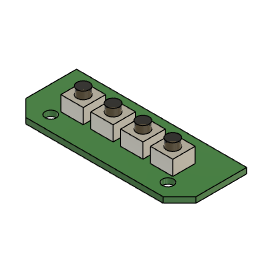
Tamabunni v1 (Autodesk Fusion 360 archive; units mm, degrees)
design "button_pad"
Autodesk Fusion 360 part; units mm, degrees
sketch "Sketch1" plane through (0, 0, 0) normal (0, 0, 1) x (1, 0, 0)
  line L0 (-22.8, 10) -> (22.8, 10)
  line L1 (22.8, 10) -> (22.8, -10)
  line L2 (22.8, -10) -> (-22.8, -10)
  line L3 (-22.8, -10) -> (-22.8, 10)
  line L4 (-22.8, 10) -> (22.8, -10) construction
  line L5 (-15, 4) -> (-9, 4)
  line L6 (-9, 4) -> (-9, -2)
  line L7 (-9, -2) -> (-15, -2)
  line L8 (-15, -2) -> (-15, 4)
  line L9 (0, 10) -> (0, -10) construction
  line L10 (-1, -2) -> (-7, -2)
  line L11 (-7, -2) -> (-7, 4)
  line L12 (-7, 4) -> (-1, 4)
  line L13 (-1, 4) -> (-1, -2)
  line L14 (7, 4) -> (1, 4)
  line L15 (1, 4) -> (1, -2)
  line L16 (1, -2) -> (7, -2)
  line L17 (7, -2) -> (7, 4)
  line L18 (15, 4) -> (9, 4)
  line L19 (9, 4) -> (9, -2)
  line L20 (15, -2) -> (15, 4)
  line L21 (9, -2) -> (15, -2)
  circle A0 centre (-15.7, -4) radius 1.5
  circle A1 centre (15.7, -4) radius 1.5
  line L22 (-15.7, -4) -> (15.7, -4) construction
  dimension "d1" = 45.6
  dimension "d2" = 20
  dimension "d3" = 6
  dimension "d4" = 6
  dimension "d5" = 2
  dimension "d6" = 1
  dimension "d7" = 6
  dimension "d33" = 7.1
  dimension "d34" = 3
  dimension "d37" = 3
  dimension "d38" = 6
  dimension "d59" = 7.1
  constraint horizontal L0
  constraint vertical L1
  constraint horizontal L2
  constraint vertical L3
  constraint midpoint origin L4
  constraint horizontal L5
  constraint vertical L6
  constraint horizontal L7
  constraint vertical L8
  constraint equal L5 L6
  constraint midpoint L0 L9.start
  constraint midpoint L2 L9.end
  constraint horizontal L12
  constraint vertical L13
  constraint horizontal L10
  constraint vertical L11
  constraint equal L12 L13
  constraint collinear L5 L12
  constraint symmetric L5.start L9 L18.start
  constraint symmetric L5.end L9 L18.end
  constraint symmetric L6.end L9 L19.end
  constraint symmetric L7.end L9 L20.start
  constraint symmetric L9 L10.start L15.end
  constraint symmetric L9 L11.end L14.start
  constraint symmetric L9 L10.end L16.end
  constraint symmetric L9 L12.end L14.end
  constraint coincident A0.centre L22.start
  constraint coincident A1.centre L22.end
  constraint horizontal L22
  measures "d1" distance of L0.start L0.end
  measures "d2" distance of L0.start L2.end
  measures "d3" distance of L5.end L6.end
  measures "d4" distance of L10.start L12.end
  measures "d5" distance of L6 L11
  measures "d6" distance of L9 L13
  measures "d7" distance of L0 L12
  measures "d33" distance of L1 A1.centre
  measures "d34" diameter of A1
  measures "d37" diameter of A0
  measures "d38" distance of L2 A1.centre
  measures "d59" distance of L3 A0.centre
extrude "Extrude7" add sketch "Sketch1" against normal blind 1.5 contours L0 L1 L2 L3 | L5 L6 L7 L8 | L10 L11 L12 L13 | L14 L15 L16 L17 | L18 L19 L20 L21
extrude "Extrude8" add sketch "Sketch1" along normal blind 4 contours L5 L6 L7 L8 | L10 L11 L12 L13 | L14 L15 L16 L17 | L18 L19 L20 L21
sketch "Sketch6" plane through (0, 0, 4) normal (0, 0, 1) x (-1, 0, 0)
  line L0 (15, 2) -> (9, 2)
  line L1 (9, 2) -> (9, -4)
  line L2 (9, -4) -> (15, -4)
  line L3 (15, -4) -> (15, 2)
  line L4 (15, -4) -> (9, 2) construction
  circle A0 centre (12, -1) radius 1.7
  dimension "d44" = 3.4
  constraint coincident L2.end L3.start
  constraint coincident L0.end L1.start
  constraint midpoint L4 A0.centre
  measures "d44" diameter of A0
sketch "Sketch7" plane through (0, 0, 4) normal (0, 0, 1) x (-1, 0, 0)
  line L0 (1, -4) -> (7, -4)
  line L1 (7, -4) -> (7, 2)
  line L2 (7, 2) -> (1, 2)
  line L3 (1, 2) -> (1, -4)
  line L4 (7, -4) -> (1, 2) construction
  circle A0 centre (4, -1) radius 1.7
  dimension "d45" = 3.4
  constraint coincident L0.end L1.start
  constraint coincident L2.end L3.start
  constraint midpoint L4 A0.centre
  measures "d45" diameter of A0
extrude "Extrude9" add sketch "Sketch6" sketch "Sketch7" along normal blind 2 contours A0 of sketch 2 contours A0
mirror "Mirror2" about plane through (0, 0, 0) normal (1, 0, 0) of "Extrude9"
sketch "Sketch8" plane through (0, 0, 0) normal (0, 0, 1) x (-1, 0, 0)
  line L0 (-9, 2) -> (-9, -4)
  line L1 (-9, -4) -> (-15, -4)
  line L2 (-15, -4) -> (-15, 2)
  line L3 (-15, 2) -> (-9, 2)
  line L4 (15, 2) -> (15, -4)
  line L5 (15, -4) -> (9, -4)
  line L6 (9, -4) -> (9, 2)
  line L7 (9, 2) -> (15, 2)
  line L8 (-7, 2) -> (-1, 2)
  line L9 (-1, 2) -> (-1, -4)
  line L10 (-1, -4) -> (-7, -4)
  line L11 (-7, -4) -> (-7, 2)
  line L12 (1, -4) -> (1, 2)
  line L13 (1, 2) -> (7, 2)
  line L14 (7, 2) -> (7, -4)
  line L15 (7, -4) -> (1, -4)
  circle A0 centre (15.7, 4) radius 1.5
  circle A1 centre (-15.7, 4) radius 1.5
  line L16 (22.8, 10) -> (-22.8, 10)
  line L17 (-22.8, 10) -> (-22.8, -10)
  line L18 (-22.8, -10) -> (22.8, -10)
  line L19 (22.8, -10) -> (22.8, 10)
  line L20 (16.3985, 10) -> (22.8, 3.5985)
  line L21 (15.7, 4) -> (19.5993, 6.7993) construction
  line L22 (0, 0) -> (0, -10) construction
  line L23 (-16.3985, 10) -> (-22.8, 3.5985)
  dimension "d51" = 45
  dimension "d52" = 4.8
  constraint coincident L16 L20.start
  constraint coincident L19 L20.end
  constraint coincident A0.centre L21.start
  constraint midpoint L20 L21.end
  constraint coincident L22.start origin
  constraint midpoint L18 L22.end
  constraint symmetric L20.start L22 L23.start
  constraint symmetric L20.end L22 L23.end
  measures "d51" angle of L19 L20
  measures "d52" distance of A0.centre L21.end
extrude "Extrude10" cut sketch "Sketch8" against normal blind 1.5 contours L16 L19 L20 | L16 L17 L23
move_face "OffsetFaces1" offset -2 1 faces at (5.4662, -10, -0.5)
extrude "Extrude1" [suppressed]
extrude "Extrude2" [suppressed]
sketch "Sketch2" plane through (0, 0, 4) normal (0, 0, 1) x (-1, 0, 0)
  line L0 (15, 2) -> (9, 2)
  line L1 (9, 2) -> (9, -4)
  line L2 (9, -4) -> (15, -4)
  line L3 (15, -4) -> (15, 2)
  circle A0 centre (12, -1) radius 2
  line L4 (15, -4) -> (9, 2) construction
  dimension "d12" = 4
  constraint coincident L2.end L3.start
  constraint coincident L0.end L1.start
  constraint midpoint A0.centre L4
  measures "d12" diameter of A0
extrude "Extrude3" [suppressed]
sketch "Sketch3" plane through (0, 0, 4) normal (0, 0, 1) x (-1, 0, 0)
  line L0 (1, -4) -> (7, -4)
  line L1 (7, -4) -> (7, 2)
  line L2 (7, 2) -> (1, 2)
  line L3 (1, 2) -> (1, -4)
  line L4 (7, -4) -> (1, 2) construction
  circle A0 centre (4, -1) radius 2
  dimension "d15" = 4
  constraint coincident L0.end L1.start
  constraint coincident L2.end L3.start
  constraint midpoint L4 A0.centre
  measures "d15" diameter of A0
extrude "Extrude4" [suppressed]
mirror "Mirror1" [suppressed]
sketch "Sketch4" plane through (0, 0, 0) normal (0, 0, 1) x (-1, 0, 0)
  line L0 (-9, 2) -> (-9, -4)
  line L1 (-9, -4) -> (-15, -4)
  line L2 (-15, -4) -> (-15, 2)
  line L3 (-15, 2) -> (-9, 2)
  line L4 (15, 2) -> (15, -4)
  line L5 (15, -4) -> (9, -4)
  line L6 (9, -4) -> (9, 2)
  line L7 (9, 2) -> (15, 2)
  line L8 (-7, 2) -> (-1, 2)
  line L9 (-1, 2) -> (-1, -4)
  line L10 (-1, -4) -> (-7, -4)
  line L11 (-7, -4) -> (-7, 2)
  line L12 (1, -4) -> (1, 2)
  line L13 (1, 2) -> (7, 2)
  line L14 (7, 2) -> (7, -4)
  line L15 (7, -4) -> (1, -4)
  line L16 (22.8, 10) -> (-22.8, 10)
  line L17 (-22.8, 10) -> (-22.8, -10)
  line L18 (-22.8, -10) -> (22.8, -10)
  line L19 (22.8, -10) -> (22.8, 10)
  circle A0 centre (-19.6, -3.8) radius 1.5
  circle A1 centre (17.3, 3.5) radius 1.5
  dimension "d20" = 3
  dimension "d21" = 3.2
  dimension "d22" = 6.2
  dimension "d23" = 3
  dimension "d24" = 6.5
  dimension "d25" = 5.5
  measures "d20" diameter of A0
  measures "d21" distance of L17 A0.centre
  measures "d22" distance of L18 A0.centre
  measures "d23" diameter of A1
  measures "d24" distance of L16 A1.centre
  measures "d25" distance of L19 A1.centre
extrude "Extrude5" [suppressed]
sketch "Sketch5" plane through (0, 0, 0) normal (0, 0, 1) x (-1, 0, 0)
  circle A0 centre (-19.6, -3.8) radius 1.5
  circle A1 centre (17.3, 3.5) radius 1.5
  line L0 (-9, 2) -> (-9, -4)
  line L1 (-9, -4) -> (-15, -4)
  line L2 (-15, -4) -> (-15, 2)
  line L3 (-15, 2) -> (-9, 2)
  line L4 (15, 2) -> (15, -4)
  line L5 (15, -4) -> (9, -4)
  line L6 (9, -4) -> (9, 2)
  line L7 (9, 2) -> (15, 2)
  line L8 (-7, 2) -> (-1, 2)
  line L9 (-1, 2) -> (-1, -4)
  line L10 (-1, -4) -> (-7, -4)
  line L11 (-7, -4) -> (-7, 2)
  line L12 (1, -4) -> (1, 2)
  line L13 (1, 2) -> (7, 2)
  line L14 (7, 2) -> (7, -4)
  line L15 (7, -4) -> (1, -4)
  line L16 (22.8, 10) -> (-22.8, 10)
  line L17 (-22.8, 10) -> (-22.8, -10)
  line L18 (-22.8, -10) -> (22.8, -10)
  line L19 (22.8, -10) -> (22.8, 10)
  line L20 (14.3, 3.2) -> (-22.8, 3.2)
  line L21 (-22.8, 3.2) -> (-22.8, 10)
  line L22 (-22.8, 10) -> (14.3, 10)
  line L23 (14.3, 10) -> (14.3, 3.2)
  dimension "d28" = 6.8
  dimension "d29" = 8.5
  constraint horizontal L20
  constraint vertical L21
  constraint horizontal L22
  constraint vertical L23
  constraint collinear L16 L22
  constraint collinear L17 L21
  measures "d28" distance of L20 L22
  measures "d29" distance of L19 L23
extrude "Extrude6" [suppressed]
equation "d22 = 4.7 mm + 1.5 mm"
